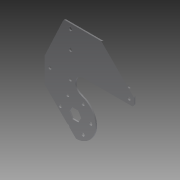
# Autodesk Inventor part: Lexan flexible Arm Mount
Saved by Autodesk Inventor 2014 (Build 180170000, 170)
## iProperties
Created: 2014-02-11
Part Number: Lexan flexible Arm Mount
Material: Polycarbonate, Clear
Document SubType Name: Modeling
Designer: Michael
Density: 1.2 g/cm^3
Appearance: Polycarbonate - Clear
Author: Michael
Autodesk Inventor part; units mm, degrees
ref_plane "YZ Plane" through (0, 0, 0) normal (1, 0, 0) x (0, 1, 0)
ref_plane "XZ Plane" through (0, 0, 0) normal (0, 1, 0) x (-1, 0, 0)
ref_plane "XY Plane" through (0, 0, 0) normal (0, 0, 1) x (1, 0, 0)
sketch "Sketch1" plane through (0, 0, 0) normal (0, 0, 1) x (1, 0, 0)
  circle A0 centre (19.05, 19.05) radius 7.9375
  line L0 (22.7162, 25.4) -> (26.3823, 19.05)
  line L1 (26.3823, 19.05) -> (22.7162, 12.7)
  line L2 (22.7162, 12.7) -> (15.3838, 12.7)
  line L3 (15.3838, 12.7) -> (11.7177, 19.05)
  line L4 (11.7177, 19.05) -> (15.3838, 25.4)
  line L5 (15.3838, 25.4) -> (22.7162, 25.4)
  circle A1 centre (0, 19.05) radius 2.0828
  line L6 (0, 19.05) -> (19.05, 19.05) construction
  circle A2 centre (9.525, 2.5522) radius 2.0828
  circle A3 centre (28.575, 2.5522) radius 2.0828
  circle A4 centre (38.1, 19.05) radius 2.0828
  circle A5 centre (28.575, 35.5478) radius 2.0828
  circle A6 centre (9.525, 35.5478) radius 2.0828
  circle A7 centre (19.05, 19.05) radius 25.4
  line L7 (19.05, -6.35) -> (-19.05, -6.35)
  line L8 (-19.05, -6.35) -> (-19.05, 57.15)
  line L9 (6.3948, 114.3) -> (92.075, 114.3)
  line L10 (92.075, 114.3) -> (92.075, 63.5)
  line L11 (92.075, 63.5) -> (29.3317, 63.5)
  line L12 (-121.3454, 55.7276) -> (199.3502, 55.7276) construction
  arc A8 (29.3317, 63.5) -> (26.369, 43.3727) centre (29.3317, 53.2183) ccw
  circle A9 centre (85.725, 69.85) radius 2.0828
  circle A10 centre (85.725, 82.55) radius 2.0828
  circle A11 centre (85.725, 95.25) radius 2.0828
  circle A12 centre (85.725, 107.95) radius 2.0828
  line L13 (29.3317, 53.2183) -> (19.05, 53.2183) construction
  line L14 (-19.05, 57.15) -> (6.3948, 114.3)
  circle A13 centre (-12.7, 53.975) radius 2.0828
  circle A14 centre (12.7, 53.975) radius 2.0828
  circle A15 centre (12.7, 85.725) radius 2.0828
  circle A16 centre (-12.7, 22.225) radius 2.0828
  circle A17 centre (12.7, 107.95) radius 2.0828
  point P0 (0, 0)
  point P1 (19.05, 44.45)
  dimension "d7" = 15.875
  dimension "d8" = 12.7
  dimension "d23" = 4.1656
  dimension "d25" = 19.05
  dimension "d26" = 0
  dimension "d29" = 360
  dimension "d41" = 50.8
  dimension "d42" = 19.05
  dimension "d43" = 19.05
  dimension "d44" = 38.1
  dimension "d55" = 73.025
  dimension "d57" = 4.1656
  dimension "d58" = 6.35
  dimension "d59" = 6.35
  dimension "d62" = 12.7
  dimension "d67" = 6.35
  dimension "d68" = 36.6776
  dimension "d69" = 50.8
  dimension "d70" = 38.1
  dimension "d71" = 114
  dimension "d72" = 57.15
  dimension "d76" = 56.3933
  dimension "d78" = 6.35
  dimension "d79" = 3.175
  dimension "d84" = 25.4
  dimension "d91" = 31.75
  dimension "d98" = 31.75
  dimension "d105" = 22.225
  constraints: 30 end point, 18 centre point, 6 horizontal, 6 point on circle, 5 vertical, 3 tangent, 2 coincident, 1 equal radius, 1 parallel, 1 perpendicular, 40 other
  measures "d7" diameter of A0
  measures "d8" distance between parallel lines of L5 L2
  measures "d23" diameter of A1
  measures "d25" distance of L6.end L6.start
  measures "d26" angle of L2 L6
  measures "d41" diameter of A7
  measures "d42" horizontal distance of A7.centre point (0, 0)
  measures "d43" horizontal distance of point (0, 0) A0.centre
  measures "d44" horizontal distance of A0.centre L7.end
  measures "d55" distance from line of L10 A0.centre
  measures "d57" diameter of A9
  measures "d58" distance from line of L11 A9.centre
  measures "d59" distance from line of L10 A9.centre
  measures "d62" distance of A9.centre A10.centre
  measures "d67" distance from line of L9 A12.centre
  measures "d68" distance from line of A0.centre L12
  measures "d69" vertical distance of A9.centre A0.centre
  measures "d70" distance from line of L8 L13.end
  measures "d71" angle of L9 L14
  measures "d72" distance from line of L8.end L9
  measures "d76" horizontal distance of A12.centre L11.end
  measures "d78" distance from line of L8 A13.centre
  measures "d79" vertical distance of L8.end A13.centre
  measures "d84" distance of A13.centre A14.centre
  measures "d91" distance of A14.centre A15.centre
  measures "d98" distance of A13.centre A16.centre
  measures "d105" distance of A15.centre A17.centre
extrude "Extrusion1" add sketch "Sketch1" along normal blind 1.5875 contours A0 | A7 | A7 L7 L8 L14 L9 L10 L11 A8
fillet "Fillet1" radius 3.175 5 edges at (6.3948, 114.3, 0.7937) (-19.05, 57.15, 0.7937) (92.075, 114.3, 0.7937) (92.075, 63.5, 0.7937) (-19.05, -6.35, 0.7937)
equation "\"d67\" = d58"
body "Solid1"
